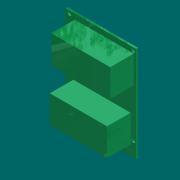
# Autodesk Inventor part: PCB
Saved by Autodesk Inventor 2020 (Build 240168000, 168)
## iProperties
Created: 2025-02-23
Part Number: PCB
Material: Plastica ABS
Document SubType Name: Modeling
Designer: Nicola Milia
Density: 1.06 g/cm^3
Appearance: Liscia - Bianco
Author: Nicola Milia
Autodesk Inventor part; units mm, degrees
ref_plane "YZ Plane" through (0, 0, 0) normal (1, 0, 0) x (0, 1, 0)
ref_plane "XZ Plane" through (0, 0, 0) normal (0, 1, 0) x (-1, 0, 0)
ref_plane "XY Plane" through (0, 0, 0) normal (0, 0, 1) x (1, 0, 0)
sketch "Schizzo1" plane through (0, 0, 0) normal (0, 0, 1) x (1, 0, 0)
  line L0 (0, 0) -> (90, 0)
  line L1 (90, 0) -> (90, -122)
  line L2 (90, -122) -> (0, -122)
  line L3 (0, -122) -> (0, 0)
  dimension "d0" = 90
  dimension "d1" = 122
  constraints: 8 end point, 2 parallel, 1 horizontal, 1 perpendicular
  measures "d0" distance of L1.end L2.end
  measures "d1" distance of L0.end L1.end
extrude "Estrusione1" add sketch "Schizzo1" along normal blind 2.5
sketch "Schizzo2" plane through (0, 0, 2.5) normal (0, 0, 1) x (1, 0, 0)
  line L0 (90, 0) -> (0, 0) projected
  line L1 (0, -122) -> (90, -122) projected
  line L2 (90, 0) -> (87, 0)
  line L3 (87, -6.7) -> (12, -6.7)
  line L4 (12, -6.7) -> (12, -41.7)
  line L5 (12, -41.7) -> (87, -41.7)
  line L6 (87, -41.7) -> (87, -6.7)
  line L7 (0, -122) -> (10, -122)
  line L8 (10, -109) -> (83, -109)
  line L9 (83, -109) -> (83, -74)
  line L10 (83, -74) -> (10, -74)
  line L11 (10, -74) -> (10, -109)
  point P0 (87, -6.7)
  dimension "d6" = 75
  dimension "d7" = 35
  dimension "d10" = 73
  dimension "d11" = 35
  constraints: 20 end point, 4 parallel, 2 horizontal, 2 perpendicular, 2 point on line
  measures "d6" distance of L5.end L4.end
  measures "d7" distance of L4.end L3.end
  measures "d10" distance of L10.end L9.end
  measures "d11" distance of L9.end L8.end
extrude "Estrusione2" add sketch "Schizzo2" along normal blind 30
sketch "Schizzo3" plane through (0, 0, 2.5) normal (0, 0, 1) x (1, 0, 0)
  line L0 (90, -122) -> (90, 0) projected
  line L1 (90, 0) -> (0, 0) projected
  line L2 (90, 0) -> (90, -6)
  line L3 (90, 0) -> (86.5, 0)
  circle A0 centre (86.5, -3.5) radius 2.5
  circle A1 centre (5, -3.5) radius 2.5
  circle A2 centre (5, -103) radius 2.5
  circle A3 centre (86.5, -103) radius 2.5
  constraints: 4 centre point, 4 end point, 2 point on line
extrude "Estrusione3" cut sketch "Schizzo3" against normal up to surface (2.5 mm away)
